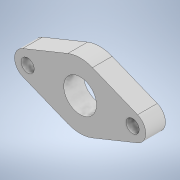
# Autodesk Inventor part: Exercício1.6
Saved by Autodesk Inventor 2022 (Build 260153000, 153)
## iProperties
Created: 2023-03-07
Part Number: Exercício1.6
Material: Genérico
Document SubType Name: Modeling
Designer: jpjoa
Density: 1 g/cm^3
Appearance: Padrão
Author: jpjoa
Autodesk Inventor part; units mm, degrees
ref_plane "YZ Plane" through (0, 0, 0) normal (1, 0, 0) x (0, 1, 0)
ref_plane "XZ Plane" through (0, 0, 0) normal (0, 1, 0) x (-1, 0, 0)
ref_plane "XY Plane" through (0, 0, 0) normal (0, 0, 1) x (1, 0, 0)
sketch "Esboço1" plane through (0, 0, 0) normal (0, 0, 1) x (1, 0, 0)
  circle A0 centre (0, 0) radius 5
  circle A1 centre (80, 0) radius 5
  circle A2 centre (40, 0) radius 12.5
  circle A3 centre (0, 0) radius 10
  circle A4 centre (40, 0) radius 25
  circle A5 centre (80, 0) radius 10
  line L0 (-3.75, 9.2702) -> (30.625, 23.1756)
  line L1 (49.375, 23.1756) -> (83.75, 9.2702)
  line L2 (49.375, -23.1756) -> (83.75, -9.2702)
  line L3 (-3.75, -9.2702) -> (30.625, -23.1756)
  dimension "d0" = 10
  dimension "d1" = 10
  dimension "d2" = 80
  dimension "d3" = 25
  dimension "d4" = 40
  dimension "d5" = 20
  dimension "d6" = 50
  dimension "d9" = 20
  constraints: 8 end point, 8 point on circle, 8 tangent, 6 centre point, 3 coincident, 3 concentric, 3 horizontal alignment
  measures "d0" diameter of A0
  measures "d1" diameter of A1
  measures "d2" distance of A1.centre point (0, 0)
  measures "d3" diameter of A2
  measures "d4" distance of A1.centre A2.centre
  measures "d5" diameter of A3
  measures "d6" diameter of A4
  measures "d9" diameter of A5
extrude "Extrusão1" add sketch "Esboço1" along normal blind 15
